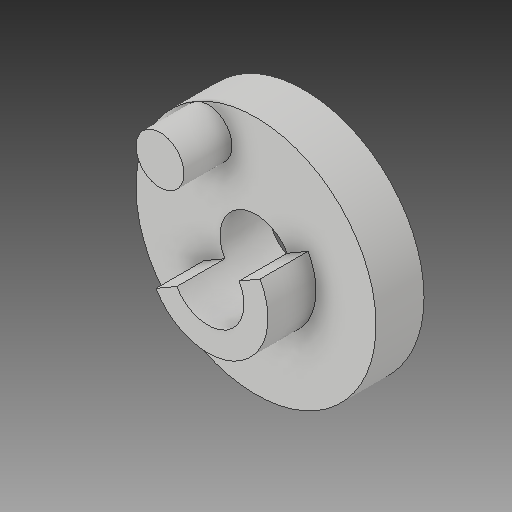
# Autodesk Inventor part: C
Saved by Autodesk Inventor 2019 (Build 230136000, 136)
## iProperties
Created: 2020-03-27
Part Number: C
Material: Generic
Document SubType Name: Modeling
Designer: Pulag
Density: 1 g/cm^3
Appearance: Default
Mass: 0.161792 g
Surface Area: 2.66323 cm^2
Volume: 0.161792 cm^3
Author: Pulag
Autodesk Inventor part; units mm, degrees
ref_plane "YZ Plane" through (0, 0, 0) normal (1, 0, 0) x (0, 1, 0)
ref_plane "XZ Plane" through (0, 0, 0) normal (0, 1, 0) x (-1, 0, 0)
ref_plane "XY Plane" through (0, 0, 0) normal (0, 0, 1) x (1, 0, 0)
sketch "Sketch1" plane through (0, 0, 0) normal (0, 0, 1) x (1, 0, 0)
  circle A0 centre (2.5, 2.5) radius 5
  circle A1 centre (0.5, 5.9641) radius 1
  circle A2 centre (2.5, 2.5) radius 2.5
  point P0 (0, 0)
  point P1 (0, 0)
  point P2 (-2.5, 2.5)
  point P3 (0, 6.8301)
  point P4 (0, -1.8301)
  point P5 (0.5, 6.9641)
  point P6 (0, 2.5)
  point P7 (2.0779, 4.9641)
  dimension "d0" = 5
  constraints: 7 point on circle, 3 centre point
  measures "d0" distance of A0.centre A0.start
sketch "Sketch2" plane through (0, 0, 0) normal (0, 0, 1) x (1, 0, 0)
  circle A0 centre (2.5, 2.5) radius 5
  circle A1 centre (0.5, 5.9641) radius 1
  circle A2 centre (2.5, 2.5) radius 2.5
  point P0 (0, 0)
  point P1 (0, 0)
  point P2 (0, 0)
  point P3 (-2.5, 2.5)
  point P4 (0, 6.8301)
  point P5 (0, -1.8301)
  point P6 (0.5, 6.9641)
  point P7 (0, 2.5)
  point P8 (2.0779, 4.9641)
  dimension "d1" = 5
  constraints: 7 point on circle, 3 centre point
  measures "d1" distance of A0.centre A0.start
extrude "Extrusion1" add sketch "Sketch1" along normal blind 2 contours A1
extrude "Extrusion2" add sketch "Sketch2" against normal blind 2 contours A1 | A0 | A2
sketch "Sketch3" plane through (2.5, 2.5, 0) normal (0, 0, 1) x (1, 0, 0)
  circle A0 centre (0, 0) radius 5
  circle A1 centre (-2, 3.4641) radius 1
  arc A2 (-2.1651, -1.25) -> (2.1651, 1.25) centre (0, 0) ccw
  circle A3 centre (0, 0) radius 5 projected
  line L0 (0, 0) -> (2.1651, 1.25)
  line L1 (0, 0) -> (-2.1651, -1.25)
  circle A4 centre (-2, 3.4641) radius 1 projected
  point P0 (-2.5, -2.5)
  point P1 (-2.5, -2.5)
  point P2 (-2.5, -2.5)
  point P3 (-2.5, -2.5)
  point P4 (-5, 0)
  point P5 (-2.5, 4.3301)
  point P6 (-2.5, -4.3301)
  point P7 (-2, 4.4641)
  point P8 (-2.5, 0)
  point P9 (-0.4221, 2.4641)
  point P10 (-2.5, 4.3301)
  dimension "d6" = 5
  constraints: 9 point on circle, 4 end point, 3 centre point, 1 point on line, 2 other
  measures "d6" distance of A0.centre A0.start
extrude "Extrusion3" add sketch "Sketch3" along normal blind 2 contours L1 L0 A2
sketch "Sketch4" plane through (2.5, 2.5, -2) normal (0, 0, -1) x (-1, 0, 0)
  line L0 (-2.1651, 1.25) -> (2.1651, -1.25) projected
  circle A0 centre (0, 0) radius 1.5
  point P0 (2.5, -2.5)
  dimension "d9" = 3
  constraints: 1 centre point, 1 midpoint
  measures "d9" diameter of A0
extrude "Extrusion4" cut sketch "Sketch4" against normal up to surface (4 mm away)
body "Solid1"
